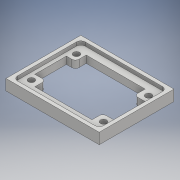
# Autodesk Inventor part: forpower
Saved by Autodesk Inventor 2019.1 (Build 231200000, 200)
## iProperties
Created: 2018-02-09
Part Number: forpower
Material: Типовые
Document SubType Name: Modeling
Designer: olege
Density: 1 g/cm^3
Appearance: По умолчанию
Author: olege
Autodesk Inventor part; units mm, degrees
ref_plane "YZ Plane" through (0, 0, 0) normal (1, 0, 0) x (0, 1, 0)
ref_plane "XZ Plane" through (0, 0, 0) normal (0, 1, 0) x (-1, 0, 0)
ref_plane "XY Plane" through (0, 0, 0) normal (0, 0, 1) x (1, 0, 0)
sketch "Эскиз1" plane through (0, 0, 0) normal (0, 0, 1) x (1, 0, 0)
  line L0 (0, 0) -> (47.7, 0)
  line L1 (47.7, 0) -> (47.7, 37.5)
  line L2 (47.7, 37.5) -> (0, 37.5)
  line L3 (0, 37.5) -> (0, 0)
  line L4 (3.85, 31.25) -> (43.85, 31.25) construction
  line L5 (43.85, 31.25) -> (43.85, 6.25) construction
  line L6 (43.85, 6.25) -> (3.85, 6.25) construction
  line L7 (3.85, 6.25) -> (3.85, 31.25) construction
  line L8 (3.85, 31.25) -> (3.85, 37.5) construction
  line L9 (3.85, 6.25) -> (3.85, 0) construction
  line L10 (3.85, 31.25) -> (0, 31.25) construction
  line L11 (43.85, 31.25) -> (47.7, 31.25) construction
  circle A0 centre (3.85, 31.25) radius 1.7
  circle A1 centre (43.85, 31.25) radius 1.7
  circle A2 centre (43.85, 6.25) radius 1.7
  circle A3 centre (3.85, 6.25) radius 1.7
  dimension "d0" = 47.7
  dimension "d1" = 37.5
  dimension "d2" = 40
  dimension "d3" = 25
  dimension "d6" = 3.4
  constraints: 24 end point, 6 point on line, 4 centre point, 4 coincident, 4 parallel, 4 perpendicular, 2 collinear, 2 horizontal
  measures "d0" distance of L2.end L1.end
  measures "d1" distance of L1.end L0.end
  measures "d2" distance of L5.end L6.end
  measures "d3" distance of L4.end L5.end
  measures "d6" diameter of A0
extrude "Выдавливание1" add sketch "Эскиз1" along normal blind 4
sketch "Эскиз2" plane through (0, 0, 4) normal (0, 0, 1) x (1, 0, 0)
  circle A0 centre (3.85, 6.25) radius 1.7 projected
  circle A1 centre (43.85, 6.25) radius 1.7 projected
  circle A2 centre (43.85, 31.25) radius 1.7 projected
  circle A3 centre (3.85, 31.25) radius 1.7 projected
  line L0 (0, 0) -> (47.7, 0) projected
  line L1 (47.7, 0) -> (47.7, 37.5) projected
  line L2 (47.7, 37.5) -> (0, 37.5) projected
  line L3 (0, 37.5) -> (0, 0) projected
  line L4 (-2, 39.5) -> (49.7, 39.5)
  line L5 (49.7, 39.5) -> (49.7, -2)
  line L6 (49.7, -2) -> (-2, -2)
  line L7 (-2, -2) -> (-2, 39.5)
  dimension "d9" = 2
  constraints: 8 end point, 3 other
  measures "d9" distance between parallel lines of L2 L4
extrude "Выдавливание2" add sketch "Эскиз2" along normal blind 2 and the other way blind 4 contours L4 L5 L6 L7
fillet "Сопряжение1" radius 2.4 4 edges at (0, 37.5, 5) (47.7, 37.5, 5) (47.7, 0, 5) (0, 0, 5)
sketch "Эскиз3" plane through (0, 0, 4) normal (0, 0, 1) x (1, 0, 0)
  line L0 (7, 33.5) -> (39.7, 33.5)
  line L1 (39.7, 4) -> (8, 4)
  line L2 (2.4, 37.5) -> (45.3, 37.5) projected
  line L3 (47.7, 35.1) -> (47.7, 2.4) projected
  line L4 (2, 27.5) -> (7, 27.5)
  line L5 (8, 10) -> (2, 10)
  line L6 (2, 10) -> (2, 27.5)
  line L7 (39.7, 27.5) -> (45.7, 27.5)
  line L8 (45.7, 27.5) -> (45.7, 10)
  line L9 (45.7, 10) -> (39.7, 10)
  line L10 (45.3, 0) -> (2.4, 0) projected
  line L11 (0, 2.4) -> (0, 35.1) projected
  line L12 (8, 4) -> (8, 10)
  line L13 (7, 27.5) -> (7, 33.5)
  line L14 (39.7, 33.5) -> (39.7, 27.5)
  line L15 (39.7, 10) -> (39.7, 4)
  point P0 (0, 0)
  dimension "d15" = 4
  dimension "d17" = 4
  dimension "d24" = 10
  dimension "d25" = 10
  dimension "d26" = 10
  dimension "d27" = 10
  dimension "d28" = 2
  dimension "d29" = 2
  dimension "d33" = 8
  dimension "d34" = 7
  dimension "d35" = 8
  dimension "d36" = 8
  constraints: 24 end point, 7 parallel, 3 horizontal, 3 perpendicular, 1 point on line
  measures "d15" distance between parallel lines of L2 L0
  measures "d17" distance between parallel lines of L10 L1
  measures "d24" distance between parallel lines of L2 L4
  measures "d25" distance between parallel lines of L10 L5
  measures "d26" distance between parallel lines of L2 L7
  measures "d27" distance between parallel lines of L10 L9
  measures "d28" distance between parallel lines of L11 L6
  measures "d29" distance between parallel lines of L3 L8
  measures "d33" distance between parallel lines of L12 L11
  measures "d34" distance between parallel lines of L11 L13
  measures "d35" distance between parallel lines of L3 L14
  measures "d36" distance between parallel lines of L3 L15
extrude "Выдавливание3" cut sketch "Эскиз3" against normal blind 10
fillet "Сопряжение2" radius 2 4 edges at (8, 10, 2) (7, 27.5, 2) (39.7, 27.5, 2) (39.7, 10, 2)
